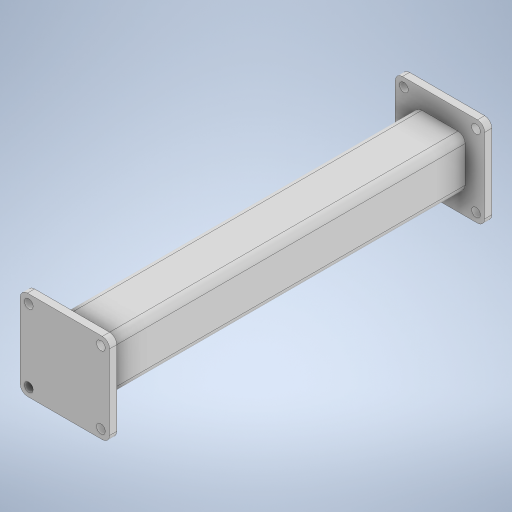
# Autodesk Inventor part: post
Saved by Autodesk Inventor 2024.3 (Build 283343000, 343)
## iProperties
Created: 2025-09-30
Part Number: post
Material: 일반
Document SubType Name: Modeling
Designer: joung
Density: 1 g/cm^3
Appearance: 기본값
Author: joung
Autodesk Inventor part; units mm, degrees
ref_plane "YZ Plane" through (0, 0, 0) normal (1, 0, 0) x (0, 1, 0)
ref_plane "XZ Plane" through (0, 0, 0) normal (0, 1, 0) x (-1, 0, 0)
ref_plane "XY Plane" through (0, 0, 0) normal (0, 0, 1) x (1, 0, 0)
sketch "스케치1" plane through (0, 0, 0) normal (0, 0, 1) x (1, 0, 0)
  line L0 (-17.5, 17.5) -> (17.5, 17.5)
  line L1 (17.5, 17.5) -> (17.5, -17.5)
  line L2 (17.5, -17.5) -> (-17.5, -17.5)
  line L3 (-17.5, -17.5) -> (-17.5, 17.5)
  line L4 (-17.5, 17.5) -> (17.5, -17.5) construction
  line L5 (17.5, 17.5) -> (-17.5, -17.5) construction
  point P0 (0, 0)
  dimension "d0" = 35
  dimension "d1" = 35
  constraints: 12 end point, 2 midpoint, 2 parallel, 1 horizontal, 1 perpendicular
  measures "d0" distance of L1.end L2.end
  measures "d1" distance of L0.end L1.end
extrude "돌출1" add sketch "스케치1" along normal blind 255
sketch "스케치2" plane through (0, 0, 255) normal (0, 0, 1) x (1, 0, 0)
  line L0 (-25, -25) -> (25, -25)
  line L1 (25, -25) -> (25, 25)
  line L2 (25, 25) -> (-25, 25)
  line L3 (-25, 25) -> (-25, -25)
  line L4 (-25, -25) -> (25, 25) construction
  line L5 (25, -25) -> (-25, 25) construction
  circle A0 centre (25, 25) radius 3.1
  circle A1 centre (-25, 25) radius 3.1
  circle A2 centre (-25, -25) radius 3.1
  circle A3 centre (25, -25) radius 3.1
  line L6 (-31, -31) -> (31, -31)
  line L7 (31, -31) -> (31, 31)
  line L8 (31, 31) -> (-31, 31)
  line L9 (-31, 31) -> (-31, -31)
  line L10 (-31, -31) -> (31, 31) construction
  line L11 (31, -31) -> (-31, 31) construction
  point P0 (0, 0)
  dimension "d4" = 50
  dimension "d5" = 50
  dimension "d6" = 6.2
  dimension "d9" = 360
  dimension "d11" = 62
  dimension "d12" = 62
  constraints: 24 end point, 4 centre point, 4 midpoint, 4 parallel, 2 horizontal, 2 perpendicular, 1 coincident, 9 other
  measures "d4" distance of L2.end L1.end
  measures "d5" distance of L1.end L0.end
  measures "d6" diameter of A0
  measures "d11" distance of L8.end L7.end
  measures "d12" distance of L7.end L6.end
extrude "돌출2" add sketch "스케치2" along normal blind 5 contours A2 L3 A1 L2 A0 L1 A3 L0 | L9 L8 L7 L6
sketch "스케치3" plane through (0, 0, 0) normal (0, 0, -1) x (-1, 0, 0)
  line L0 (-31, -31) -> (31, -31)
  line L1 (31, -31) -> (31, 31)
  line L2 (31, 31) -> (-31, 31)
  line L3 (-31, 31) -> (-31, -31)
  line L4 (-31, -31) -> (31, 31) construction
  line L5 (31, -31) -> (-31, 31) construction
  circle A0 centre (25, 25) radius 3.1 projected
  circle A1 centre (25, 25) radius 3.1
  circle A2 centre (-25, 25) radius 3.1
  circle A3 centre (-25, -25) radius 3.1
  circle A4 centre (25, -25) radius 3.1
  point P0 (0, 0)
  dimension "d17" = 360
  constraints: 12 end point, 4 centre point, 2 midpoint, 2 parallel, 1 coincident, 1 horizontal, 1 perpendicular, 9 other
extrude "돌출3" add sketch "스케치3" along normal blind 5
fillet "모깎기1" radius 5 12 edges at (17.5, 17.5, 127.5) (17.5, -17.5, 127.5) (-17.5, 17.5, 127.5) (31, 31, -2.5) (31, -31, -2.5) (-17.5, -17.5, 127.5) (-31, -31, -2.5) (-31, 31, -2.5) (-31, -31, 257.5) (-31, 31, 257.5) (31, -31, 257.5) (31, 31, 257.5)
